Autodesk Fusion 360 part; units mm, degrees
(part 2 of 3)
sketch "Sketch24" plane through (2.9845, 0, 0) normal (1, 0, 0) x (0, 0, -1)
  circle A0 centre (17.3736, 285.75) radius 11.1125
  circle A1 centre (-17.3736, 285.75) radius 11.1125
  arc A2 (-19.05, 304.8) -> (-31.75, 292.1) centre (-19.05, 292.1) ccw
  line L0 (-31.75, 292.1) -> (-31.75, 254)
  line L1 (-31.75, 254) -> (-38.1, 254)
  line L2 (-38.1, 254) -> (-38.1, 0)
  line L3 (-38.1, 0) -> (-88.9, 0)
  line L4 (-88.9, 0) -> (-88.9, 5.969)
  line L5 (-88.9, 5.969) -> (-114.3, 5.969)
  line L6 (-114.3, 5.969) -> (-114.3, -6.35)
  arc A3 (-114.3, -6.35) -> (-101.6, -19.05) centre (-101.6, -6.35) ccw
  line L7 (-101.6, -19.05) -> (101.6, -19.05)
  arc A4 (101.6, -19.05) -> (114.3, -6.35) centre (101.6, -6.35) ccw
  line L8 (114.3, -6.35) -> (114.3, 5.969)
  line L9 (114.3, 5.969) -> (88.9, 5.969)
  line L10 (88.9, 5.969) -> (88.9, 0)
  line L11 (88.9, 0) -> (38.1, 0)
  line L12 (38.1, 0) -> (38.1, 254)
  line L13 (38.1, 254) -> (31.75, 254)
  line L14 (31.75, 254) -> (31.75, 292.1)
  arc A5 (31.75, 292.1) -> (19.05, 304.8) centre (19.05, 292.1) ccw
  line L15 (19.05, 304.8) -> (2.9845, 304.8)
  line L16 (2.9845, 304.8) -> (2.9845, -9.525)
  line L17 (2.9845, -9.525) -> (-2.9845, -9.525)
  line L18 (-2.9845, -9.525) -> (-2.9845, 304.8)
  line L19 (-2.9845, 304.8) -> (-19.05, 304.8)
  line L20 (2.9845, 304.8) -> (31.7627, 304.8) construction
  line L21 (31.7627, 304.8) -> (31.7627, 228.6) construction
  line L22 (31.7627, 228.6) -> (31.7627, 203.2) construction
  line L23 (31.7627, 203.2) -> (31.7627, 177.8) construction
  line L24 (31.7627, 177.8) -> (31.7627, 152.4) construction
  line L25 (31.7627, 152.4) -> (31.7627, 127) construction
  line L26 (31.7627, 127) -> (31.75, 101.6) construction
  line L27 (31.7627, 228.6) -> (19.0627, 228.6)
  line L28 (19.0627, 228.6) -> (19.0627, 222.631)
  line L29 (19.0627, 222.631) -> (31.7627, 222.631)
  line L30 (31.7627, 222.631) -> (31.7627, 228.6)
  line L31 (31.7627, 177.8) -> (19.0627, 177.8)
  line L32 (19.0627, 177.8) -> (19.0627, 171.831)
  line L33 (19.0627, 171.831) -> (31.7627, 171.831)
  line L34 (31.7627, 171.831) -> (31.7627, 177.8)
  line L35 (31.7627, 203.2) -> (19.0627, 203.2)
  line L36 (19.0627, 203.2) -> (19.0627, 197.231)
  line L37 (19.0627, 197.231) -> (31.7627, 197.231)
  line L38 (31.7627, 197.231) -> (31.7627, 203.2)
  line L39 (31.7627, 152.4) -> (19.0627, 152.4)
  line L40 (19.0627, 152.4) -> (19.0627, 146.431)
  line L41 (19.0627, 146.431) -> (31.7627, 146.431)
  line L42 (31.7627, 146.431) -> (31.7627, 152.4)
  line L43 (31.7627, 127) -> (19.0627, 127)
  line L44 (19.0627, 127) -> (19.0627, 121.031)
  line L45 (19.0627, 121.031) -> (31.7627, 121.031)
  line L46 (31.7627, 121.031) -> (31.7627, 127)
  line L47 (31.75, 101.6) -> (19.05, 101.6)
  line L48 (19.05, 101.6) -> (19.05, 95.631)
  line L49 (19.05, 95.631) -> (31.75, 95.631)
  line L50 (31.75, 95.631) -> (31.75, 101.6)
  dimension "d155" = 28.7782
  dimension "d156" = 76.2
  dimension "d157" = 25.4
  dimension "d158" = 25.4
  dimension "d159" = 25.4
  dimension "d160" = 25.4
  dimension "d161" = 25.4
  dimension "d162" = 12.7
  dimension "d163" = 5.969
  dimension "d164" = 12.7
  dimension "d165" = 5.969
  dimension "d166" = 12.7
  dimension "d167" = 5.969
  dimension "d168" = 12.7
  dimension "d169" = 5.969
  dimension "d170" = 12.7
  dimension "d171" = 5.969
  dimension "d172" = 12.7
  dimension "d173" = 5.969
  constraint coincident L15.end L16.start
  constraint perpendicular L16 L20
  constraint perpendicular L20 L21
  constraint parallel L14 L22
  constraint parallel L14 L23
  constraint parallel L14 L24
  constraint parallel L16 L25
  constraint coincident L14 L26.end
  constraint horizontal L27
  constraint vertical L28
  constraint horizontal L29
  constraint vertical L30
  constraint horizontal L31
  constraint vertical L32
  constraint horizontal L33
  constraint vertical L34
  constraint horizontal L35
  constraint vertical L36
  constraint horizontal L37
  constraint vertical L38
  constraint horizontal L39
  constraint vertical L40
  constraint horizontal L41
  constraint vertical L42
  constraint horizontal L43
  constraint vertical L44
  constraint horizontal L45
  constraint vertical L46
  constraint horizontal L47
  constraint vertical L48
  constraint horizontal L49
  constraint vertical L50
  measures "d155" distance of L15.end L20.end
  measures "d156" distance of L20.end L21.end
  measures "d157" distance of L21.end L22.end
  measures "d158" distance of L22.end L23.end
  measures "d159" distance of L23.end L24.end
  measures "d160" distance of L24.end L25.end
  measures "d161" distance of L25.end L26.end
  measures "d162" distance of L21.end L27.end
  measures "d163" distance of L21.end L29.end
  measures "d164" distance of L23.end L31.end
  measures "d165" distance of L23.end L33.end
  measures "d166" distance of L22.end L35.end
  measures "d167" distance of L22.end L37.end
  measures "d168" distance of L24.end L39.end
  measures "d169" distance of L24.end L41.end
  measures "d170" distance of L25.end L43.end
  measures "d171" distance of L25.end L45.end
  measures "d172" distance of L26.end L47.end
  measures "d173" distance of L26.end L49.end
sketch "Sketch25" plane through (0, 0, 0) normal (0, 1, 0) x (1, 0, 0)
  line L0 (31.369, -190.5) -> (31.369, -279.4)
  line L1 (31.369, -279.4) -> (0, -279.4)
  line L2 (0, -279.4) -> (0, -190.5)
  line L3 (12.7127, -279.4) -> (18.6817, -279.4)
  line L4 (18.6817, -203.2) -> (12.7127, -203.2)
  arc A0 (31.369, -190.5) -> (0, -190.5) centre (15.6845, -190.5) ccw
  line L5 (0, -279.4) -> (12.7, -279.4) construction
  line L6 (12.7, -279.4) -> (18.669, -279.4)
  line L7 (18.669, -279.4) -> (18.669, -203.2)
  line L8 (18.669, -203.2) -> (12.7, -203.2)
  line L9 (12.7, -203.2) -> (12.7, -279.4)
  arc A1 (0, -203.2) -> (0, -190.5) centre (-6.35, -196.85) ccw
  line L10 (0, -190.5) -> (0, -196.85) construction
  line L11 (0, -196.85) -> (2.6303, -196.85) construction
  line L12 (31.369, -190.5) -> (31.369, -196.85) construction
  line L13 (31.369, -196.85) -> (28.7274, -196.85) construction
  arc A2 (31.369, -190.5) -> (31.369, -203.2) centre (37.6804, -196.85) ccw
  line L14 (18.6817, -203.2) -> (18.6817, -225.2472) construction
  dimension "d176" = 31.369
  dimension "d177" = 88.9
  dimension "d180" = 76.2
  dimension "d185" = 12.7
  dimension "d186" = 5.969
  dimension "d187" = 76.2
  dimension "d189" = 12.7
  dimension "d190" = 6.35
  dimension "d191" = 6.35
  dimension "d192" = 2.6416
  dimension "d193" = 12.7
  dimension "d194" = 22.0472
  constraint vertical L0
  constraint horizontal L1
  constraint vertical L2
  constraint horizontal L3
  constraint horizontal L4
  constraint tangent L0 A0
  constraint perpendicular L2 L5
  constraint horizontal L6
  constraint vertical L7
  constraint horizontal L8
  constraint vertical L9
  constraint coincident L2 A1.start
  constraint parallel L2 L10
  constraint midpoint A1 L11.end
  constraint perpendicular L11 L12
  constraint perpendicular L12 L13
  constraint coincident L13.end A2
  constraint coincident L0 A2.end
  constraint perpendicular L8 L14
  measures "d176" distance of L2.end L0.start
  measures "d177" distance of L2.end L1.end
  measures "d180" distance of L3.start L4.end
  measures "d185" distance of L1.end L5.end
  measures "d186" distance of L5.end L6.end
  measures "d187" distance of L5.end L8.end
  measures "d189" distance of L2.end A1.start
  measures "d190" distance of L2.end L10.end
  measures "d191" distance of L0.start L12.end
  measures "d192" distance of L12.end L13.end
  measures "d193" distance of L0.start A2.end
  measures "d194" distance of L4.start L14.end
sketch "Sketch26" plane through (-2.9845, 0, 0) normal (-1, 0, 0) x (0, 0, 1)
  line L0 (-31.75, 254) -> (-38.1, 254)
  line L1 (-38.1, 254) -> (-38.1, 0)
  line L2 (-38.1, 0) -> (-88.9, 0)
  line L3 (-88.9, 0) -> (-88.9, 5.969)
  line L4 (-88.9, 5.969) -> (-114.3, 5.969)
  line L5 (-114.3, 5.969) -> (-114.3, -6.35)
  arc A0 (-114.3, -6.35) -> (-101.6, -19.05) centre (-101.6, -6.35) ccw
  line L6 (-101.6, -19.05) -> (101.6, -19.05)
  arc A1 (101.6, -19.05) -> (114.3, -6.35) centre (101.6, -6.35) ccw
  line L7 (114.3, -6.35) -> (114.3, 5.969)
  line L8 (114.3, 5.969) -> (88.9, 5.969)
  line L9 (88.9, 5.969) -> (88.9, 0)
  line L10 (88.9, 0) -> (38.1, 0)
  line L11 (38.1, 0) -> (38.1, 254)
  line L12 (38.1, 254) -> (31.75, 254)
  line L13 (31.75, 254) -> (31.75, 292.1)
  arc A2 (31.75, 292.1) -> (19.05, 304.8) centre (19.05, 292.1) ccw
  line L14 (19.05, 304.8) -> (2.9845, 304.8)
  line L15 (2.9845, 304.8) -> (2.9845, -9.525)
  line L16 (2.9845, -9.525) -> (-2.9845, -9.525)
  line L17 (-2.9845, -9.525) -> (-2.9845, 304.8)
  line L18 (-2.9845, 304.8) -> (-19.05, 304.8)
  arc A3 (-19.05, 304.8) -> (-31.75, 292.1) centre (-19.05, 292.1) ccw
  line L19 (-31.75, 292.1) -> (-31.75, 254)
  circle A4 centre (17.3736, 285.75) radius 11.1125
  circle A5 centre (-17.3736, 285.75) radius 11.1125
sketch "Sketch27" plane through (0, 0, 2.9845) normal (0, 0, 1) x (1, 0, 0)
  circle A0 centre (17.3609, 285.75) radius 11.1125
  circle A1 centre (-17.3609, 285.75) radius 11.1125
  arc A2 (-19.05, 304.8) -> (-31.75, 292.1) centre (-19.05, 292.1) ccw
  line L0 (-31.75, 292.1) -> (-31.75, 254)
  line L1 (-31.75, 254) -> (-38.1, 254)
  line L2 (-38.1, 254) -> (-38.1, 0)
  line L3 (-38.1, 0) -> (-88.9, 0)
  line L4 (-88.9, 0) -> (-88.9, 5.969)
  line L5 (-88.9, 5.969) -> (-114.3, 5.969)
  line L6 (-114.3, 5.969) -> (-114.3, -6.35)
  arc A3 (-114.3, -6.35) -> (-101.6, -19.05) centre (-101.6, -6.35) ccw
  line L7 (-101.6, -19.05) -> (-2.9845, -19.05)
  line L8 (-2.9845, -19.05) -> (-2.9845, -9.525)
  line L9 (-2.9845, -9.525) -> (2.9845, -9.525)
  line L10 (2.9845, -9.525) -> (2.9845, -19.05)
  line L11 (2.9845, -19.05) -> (101.6, -19.05)
  arc A4 (101.6, -19.05) -> (114.3, -6.35) centre (101.6, -6.35) ccw
  line L12 (114.3, -6.35) -> (114.3, 5.969)
  line L13 (114.3, 5.969) -> (88.9, 5.969)
  line L14 (88.9, 5.969) -> (88.9, 0)
  line L15 (88.9, 0) -> (38.1, 0)
  line L16 (38.1, 0) -> (38.1, 254)
  line L17 (38.1, 254) -> (31.75, 254)
  line L18 (31.75, 254) -> (31.75, 292.1)
  arc A5 (31.75, 292.1) -> (19.05, 304.8) centre (19.05, 292.1) ccw
  line L19 (19.05, 304.8) -> (-19.05, 304.8)
sketch "Sketch28" plane through (0, 5.969, 0) normal (0, 1, 0) x (-1, 0, 0)
  arc A0 (-495.3, 367.5922) -> (-596.1922, 266.7) centre (-482.6, 254) ccw
  line L0 (-596.1922, 266.7) -> (-602.5797, 266.7)
  arc A1 (-495.3, 373.9797) -> (-602.5797, 266.7) centre (-482.6, 254) ccw
  line L1 (-495.3, 373.9797) -> (-495.3, 367.5922)
  arc A2 (-469.9, 166.0118) -> (-394.6118, 241.3) centre (-482.6, 254) ccw
  line L2 (-394.6118, 241.3) -> (-388.2005, 241.3)
  arc A3 (-469.9, 159.6005) -> (-388.2005, 241.3) centre (-482.6, 254) ccw
  line L3 (-469.9, 159.6005) -> (-469.9, 166.0118)
  arc A4 (-420.383, 266.7) -> (-469.9, 316.217) centre (-482.6, 254) ccw
  line L4 (-469.9, 316.217) -> (-469.9, 322.6857)
  arc A5 (-413.9142, 266.7) -> (-469.9, 322.6857) centre (-482.6, 254) ccw
  line L5 (-413.9142, 266.7) -> (-420.383, 266.7)
  arc A6 (-469.9, 191.783) -> (-420.383, 241.3) centre (-482.6, 254) ccw
  line L6 (-420.383, 241.3) -> (-413.9142, 241.3)
  arc A7 (-469.9, 185.3142) -> (-413.9142, 241.3) centre (-482.6, 254) ccw
  line L7 (-469.9, 185.3142) -> (-469.9, 191.783)
  arc A8 (-394.6118, 266.7) -> (-469.9, 341.9882) centre (-482.6, 254) ccw
  line L8 (-469.9, 341.9882) -> (-469.9, 348.3995)
  arc A9 (-388.2005, 266.7) -> (-469.9, 348.3995) centre (-482.6, 254) ccw
  line L9 (-388.2005, 266.7) -> (-394.6118, 266.7)
  arc A10 (-469.9, 140.4077) -> (-369.0077, 241.3) centre (-482.6, 254) ccw
  line L10 (-369.0077, 241.3) -> (-362.6203, 241.3)
  arc A11 (-469.9, 134.0203) -> (-362.6203, 241.3) centre (-482.6, 254) ccw
  line L11 (-469.9, 134.0203) -> (-469.9, 140.4077)
  arc A12 (-369.0077, 266.7) -> (-469.9, 367.5922) centre (-482.6, 254) ccw
  line L12 (-469.9, 367.5922) -> (-469.9, 373.9797)
  arc A13 (-362.6203, 266.7) -> (-469.9, 373.9797) centre (-482.6, 254) ccw
  line L13 (-362.6203, 266.7) -> (-369.0077, 266.7)
  arc A14 (-570.5882, 241.3) -> (-495.3, 166.0118) centre (-482.6, 254) ccw
  line L14 (-495.3, 166.0118) -> (-495.3, 159.6005)
  arc A15 (-576.9995, 241.3) -> (-495.3, 159.6005) centre (-482.6, 254) ccw
  line L15 (-576.9995, 241.3) -> (-570.5882, 241.3)
  arc A16 (-495.3, 316.217) -> (-544.817, 266.7) centre (-482.6, 254) ccw
  line L16 (-544.817, 266.7) -> (-551.2857, 266.7)
  arc A17 (-495.3, 322.6857) -> (-551.2857, 266.7) centre (-482.6, 254) ccw
  line L17 (-495.3, 322.6857) -> (-495.3, 316.217)
  arc A18 (-544.817, 241.3) -> (-495.3, 191.783) centre (-482.6, 254) ccw
  line L18 (-495.3, 191.783) -> (-495.3, 185.3142)
  arc A19 (-551.2857, 241.3) -> (-495.3, 185.3142) centre (-482.6, 254) ccw
  line L19 (-551.2857, 241.3) -> (-544.817, 241.3)
  arc A20 (-495.3, 341.9882) -> (-570.5882, 266.7) centre (-482.6, 254) ccw
  line L20 (-570.5882, 266.7) -> (-576.9995, 266.7)
  arc A21 (-495.3, 348.3995) -> (-576.9995, 266.7) centre (-482.6, 254) ccw
  line L21 (-495.3, 348.3995) -> (-495.3, 341.9882)
  arc A22 (-596.1922, 241.3) -> (-495.3, 140.4077) centre (-482.6, 254) ccw
  line L22 (-495.3, 140.4077) -> (-495.3, 134.0203)
  arc A23 (-602.5797, 241.3) -> (-495.3, 134.0203) centre (-482.6, 254) ccw
  line L23 (-602.5797, 241.3) -> (-596.1922, 241.3)
  line L24 (-485.5845, 251.0155) -> (-514.35, 251.0155)
  line L25 (-514.35, 251.0155) -> (-514.35, 256.9845)
  line L26 (-514.35, 256.9845) -> (-485.5845, 256.9845)
  line L27 (-485.5845, 256.9845) -> (-485.5845, 285.75)
  line L28 (-485.5845, 285.75) -> (-479.6155, 285.75)
  line L29 (-479.6155, 285.75) -> (-479.6155, 256.9845)
  line L30 (-479.6155, 256.9845) -> (-450.85, 256.9845)
  line L31 (-450.85, 256.9845) -> (-450.85, 251.0155)
  line L32 (-450.85, 251.0155) -> (-479.6155, 251.0155)
  line L33 (-479.6155, 251.0155) -> (-479.6155, 222.25)
  line L34 (-479.6155, 222.25) -> (-485.5845, 222.25)
  line L35 (-485.5845, 222.25) -> (-485.5845, 251.0155)
  circle A24 centre (-482.6, 254) radius 152.4
  line L36 (-479.6155, 251.0155) -> (-457.1649, 228.5648) construction
  line L37 (-485.5845, 256.9845) -> (-508.0351, 279.4351) construction
  line L38 (-485.5845, 251.0155) -> (-508.0351, 228.5649) construction
  line L39 (-485.5845, 251.0155) -> (-453.8345, 251.0155) construction
  line L40 (-479.6155, 256.9845) -> (-457.1649, 279.4351) construction
  line L41 (-479.6155, 256.9845) -> (-447.8655, 256.9845) construction
  line L42 (-485.5845, 222.25) -> (-485.5845, 215.265)
  line L43 (-450.85, 251.0155) -> (-449.58, 251.0155)
  line L44 (-449.58, 251.0155) -> (-442.595, 251.0155)
  line L45 (-479.6155, 285.75) -> (-479.6155, 292.735)
  line L46 (-514.35, 256.9845) -> (-521.335, 256.9845)
  line L47 (-514.35, 251.0155) -> (-511.175, 251.0155)
  line L48 (-485.5845, 285.75) -> (-485.5845, 282.575)
  line L49 (-450.85, 256.9845) -> (-454.025, 256.9845)
  line L50 (-479.6155, 222.25) -> (-479.6155, 225.425)
  arc A25 (-479.6155, 225.425) -> (-442.595, 251.0155) centre (-472.206, 254.2792) ccw
  arc A26 (-511.175, 251.0155) -> (-485.5845, 215.265) centre (-484.108, 243.3561) ccw
  arc A27 (-485.5845, 282.575) -> (-521.335, 256.9845) centre (-493.2439, 255.508) ccw
  arc A28 (-454.025, 256.9845) -> (-479.6155, 292.735) centre (-481.092, 264.6439) ccw
  line L51 (-442.595, 251.0155) -> (-442.595, 256.9845)
  line L52 (-442.595, 256.9845) -> (-454.025, 256.9845)
  line L53 (-479.6155, 292.735) -> (-485.5845, 292.735)
  line L54 (-485.5845, 292.735) -> (-485.5845, 282.575)
  line L55 (-521.335, 256.9845) -> (-521.335, 251.0155)
  line L56 (-521.335, 251.0155) -> (-511.175, 251.0155)
  line L57 (-485.5845, 215.265) -> (-479.6155, 215.265)
  line L58 (-479.6155, 215.265) -> (-479.6155, 225.425)
  dimension "d314" = 31.75
  dimension "d315" = 31.75
  dimension "d316" = 135
  dimension "d317" = 31.75
  dimension "d320" = 45
  dimension "d321" = 31.75
  dimension "d327" = 6.985
  dimension "d328" = 6.985
  dimension "d329" = 6.985
  dimension "d330" = 6.985
  dimension "d331" = 3.175
  dimension "d332" = 3.175
  dimension "d333" = 3.175
  dimension "d334" = 3.175
  dimension "d335" = 5.969
  dimension "d336" = 5.969
  constraint coincident L29.end L30.start
  constraint coincident L32.end L33.start
  constraint coincident L26.end L27.start
  constraint horizontal L39
  constraint coincident L24.start L35.end
  constraint horizontal L41
  constraint coincident L34.end L35.start
  constraint perpendicular L34 L42
  constraint coincident L31.end L32.start
  constraint perpendicular L31 L43
  constraint perpendicular L31 L44
  constraint coincident L28.end L29.start
  constraint perpendicular L28 L45
  constraint coincident L25.end L26.start
  constraint perpendicular L25 L46
  constraint coincident L24.end L25.start
  constraint perpendicular L25 L47
  constraint coincident L27.end L28.start
  constraint perpendicular L28 L48
  constraint coincident L30.end L31.start
  constraint perpendicular L31 L49
  constraint coincident L33.end L34.start
  constraint perpendicular L34 L50
  constraint coincident L36.end A25
  constraint coincident L38.end A26
  constraint coincident L37.end A27
  constraint coincident L40.end A28
  constraint perpendicular L44 L51
  constraint perpendicular L45 L53
  constraint perpendicular L53 L54
  constraint perpendicular L46 L55
  constraint perpendicular L55 L56
  constraint perpendicular L42 L57
  measures "d314" distance of L32.end L36.end
  measures "d315" distance of L26.end L37.end
  measures "d316" angle of L38 L39
  measures "d317" distance of L24.start L38.end
  measures "d320" angle of L40 L41
  measures "d321" distance of L29.end L40.end
  measures "d327" distance of L34.end L42.end
  measures "d328" distance of L43.end L44.end
  measures "d329" distance of L28.end L45.end
  measures "d330" distance of L25.end L46.end
  measures "d331" distance of L24.end L47.end
  measures "d332" distance of L27.end L48.end
  measures "d333" distance of L30.end L49.end
  measures "d334" distance of L33.end L50.end
  measures "d335" distance of L44.end L51.end
  measures "d336" distance of L42.end L57.end
extrude "Extrude3'''" cut sketch "Sketch28" against normal up to surface (5.969 mm away) contours L24 L35 L42 A26 | L34 L42 L57 L58 | L25 L46 L55 L56 | L26 L27 L46 A27 | L32 L33 L43 L44 A25 | L31 L43 L44 L51 L52 | L28 L45 L53 L54 | L29 L30 L45 A28 bodies 6 in component "Component'''"
extrude "Extrude2''''" cut sketch "Sketch28" against normal up to surface (5.969 mm away) contours L24 L25 L26 L27 L28 L29 L30 L31 L32 L33 L34 L35 L47 L48 L49 L50 L52 L54 L56 L58 | L28 L45 L53 L54 | L29 L30 L45 A28 bodies 6 in component "Component'''"
extrude "Extrude1''''" cut sketch "Sketch28" against normal up to surface (5.969 mm away) contours L24 L35 L42 A26 | L24 L25 L26 L27 L28 L29 L30 L31 L32 L33 L34 L35 L47 L48 L49 L50 L52 L54 L56 L58 | L26 L27 L46 A27 | L32 L33 L43 L44 A25 | L29 L30 L45 A28 bodies 6 in component "Component'''"
sketch "Sketch29" plane through (0, 0, 2.9845) normal (0, 0, 1) x (1, 0, 0)
  circle A0 centre (17.3609, 285.75) radius 11.1125
  circle A1 centre (-17.3609, 285.75) radius 11.1125
  arc A2 (-19.05, 304.8) -> (-31.75, 292.1) centre (-19.05, 292.1) ccw
  line L0 (-31.75, 292.1) -> (-31.75, 254)
  line L1 (-31.75, 254) -> (-38.1, 254)
  line L2 (-38.1, 254) -> (-38.1, 0)
  line L3 (-38.1, 0) -> (-88.9, 0)
  line L4 (-88.9, 0) -> (-88.9, 5.969)
  line L5 (-88.9, 5.969) -> (-114.3, 5.969)
  line L6 (-114.3, 5.969) -> (-114.3, -6.35)
  arc A3 (-114.3, -6.35) -> (-101.6, -19.05) centre (-101.6, -6.35) ccw
  line L7 (-101.6, -19.05) -> (-2.9845, -19.05)
  line L8 (-2.9845, -19.05) -> (-2.9845, -9.525)
  line L9 (-2.9845, -9.525) -> (2.9845, -9.525)
  line L10 (2.9845, -9.525) -> (2.9845, -19.05)
  line L11 (2.9845, -19.05) -> (101.6, -19.05)
  arc A4 (101.6, -19.05) -> (114.3, -6.35) centre (101.6, -6.35) ccw
  line L12 (114.3, -6.35) -> (114.3, 5.969)
  line L13 (114.3, 5.969) -> (88.9, 5.969)
  line L14 (88.9, 5.969) -> (88.9, 0)
  line L15 (88.9, 0) -> (38.1, 0)
  line L16 (38.1, 0) -> (38.1, 254)
  line L17 (38.1, 254) -> (31.75, 254)
  line L18 (31.75, 254) -> (31.75, 292.1)
  arc A5 (31.75, 292.1) -> (19.05, 304.8) centre (19.05, 292.1) ccw
  line L19 (19.05, 304.8) -> (-19.05, 304.8)
  line L20 (38.1, 254) -> (38.1, 228.6) construction
  line L21 (38.1, 228.6) -> (38.1, 203.2) construction
  line L22 (38.1, 203.2) -> (38.1, 177.8) construction
  line L23 (38.1, 177.8) -> (38.1, 152.4) construction
  line L24 (38.1, 152.4) -> (38.1, 127) construction
  line L25 (38.1, 127) -> (38.1, 101.6) construction
  line L26 (38.1, 101.6) -> (38.1, 76.2) construction
  line L27 (38.1, 76.2) -> (38.1, 50.8) construction
  line L28 (-38.1, 254) -> (-38.1, 228.6) construction
  line L29 (-38.1, 228.6) -> (-38.1, 203.2) construction
  line L30 (-38.1, 203.2) -> (-38.1, 177.8) construction
  line L31 (-38.1, 177.8) -> (-38.1, 152.4) construction
  line L32 (-38.1, 152.4) -> (-38.1, 127) construction
  line L33 (-38.1, 127) -> (-38.1, 101.6) construction
  line L34 (-38.1, 101.6) -> (-38.1, 76.2) construction
  line L35 (-38.1, 76.2) -> (-38.1, 50.8) construction
  line L36 (-38.1, 228.6) -> (-32.131, 228.6)
  line L37 (-32.131, 228.6) -> (-32.131, 222.631)
  line L38 (-32.131, 222.631) -> (-38.1, 222.631)
  line L39 (-38.1, 222.631) -> (-38.1, 228.6)
  line L40 (-38.1, 203.2) -> (-32.131, 203.2)
  line L41 (-32.131, 203.2) -> (-32.131, 197.231)
  line L42 (-32.131, 197.231) -> (-38.1, 197.231)
  line L43 (-38.1, 197.231) -> (-38.1, 203.2)
  line L44 (-38.1, 177.8) -> (-32.131, 177.8)
  line L45 (-32.131, 177.8) -> (-32.131, 171.831)
  line L46 (-32.131, 171.831) -> (-38.1, 171.831)
  line L47 (-38.1, 171.831) -> (-38.1, 177.8)
  line L48 (-38.1, 152.4) -> (-32.131, 152.4)
  line L49 (-32.131, 152.4) -> (-32.131, 146.431)
  line L50 (-32.131, 146.431) -> (-38.1, 146.431)
  line L51 (-38.1, 146.431) -> (-38.1, 152.4)
  line L52 (-38.1, 127) -> (-32.131, 127)
  line L53 (-32.131, 127) -> (-32.131, 121.031)
  line L54 (-32.131, 121.031) -> (-38.1, 121.031)
  line L55 (-38.1, 121.031) -> (-38.1, 127)
  line L56 (-38.1, 101.6) -> (-32.131, 101.6)
  line L57 (-32.131, 101.6) -> (-32.131, 95.631)
  line L58 (-32.131, 95.631) -> (-38.1, 95.631)
  line L59 (-38.1, 95.631) -> (-38.1, 101.6)
  line L60 (-38.1, 76.2) -> (-32.131, 76.2)
  line L61 (-32.131, 76.2) -> (-32.131, 70.231)
  line L62 (-32.131, 70.231) -> (-38.1, 70.231)
  line L63 (-38.1, 70.231) -> (-38.1, 76.2)
  line L64 (-38.1, 50.8) -> (-32.131, 50.8)
  line L65 (-32.131, 50.8) -> (-32.131, 44.831)
  line L66 (-32.131, 44.831) -> (-38.1, 44.831)
  line L67 (-38.1, 44.831) -> (-38.1, 50.8)
  line L68 (38.1, 50.8) -> (32.131, 50.8)
  line L69 (32.131, 50.8) -> (32.131, 44.831)
  line L70 (32.131, 44.831) -> (38.1, 44.831)
  line L71 (38.1, 44.831) -> (38.1, 50.8)
  line L72 (38.1, 76.2) -> (32.131, 76.2)
  line L73 (32.131, 76.2) -> (32.131, 70.231)
  line L74 (32.131, 70.231) -> (38.1, 70.231)
  line L75 (38.1, 70.231) -> (38.1, 76.2)
  line L76 (38.1, 101.6) -> (32.131, 101.6)
  line L77 (32.131, 101.6) -> (32.131, 95.631)
  line L78 (32.131, 95.631) -> (38.1, 95.631)
  line L79 (38.1, 95.631) -> (38.1, 101.6)
  line L80 (38.1, 127) -> (32.131, 127)
  line L81 (32.131, 127) -> (32.131, 121.031)
  line L82 (32.131, 121.031) -> (38.1, 121.031)
  line L83 (38.1, 121.031) -> (38.1, 127)
  line L84 (38.1, 152.4) -> (32.131, 152.4)
  line L85 (32.131, 152.4) -> (32.131, 146.431)
  line L86 (32.131, 146.431) -> (38.1, 146.431)
  line L87 (38.1, 146.431) -> (38.1, 152.4)
  line L88 (38.1, 177.8) -> (32.131, 177.8)
  line L89 (32.131, 177.8) -> (32.131, 171.831)
  line L90 (32.131, 171.831) -> (38.1, 171.831)
  line L91 (38.1, 171.831) -> (38.1, 177.8)
  line L92 (38.1, 203.2) -> (32.131, 203.2)
  line L93 (32.131, 203.2) -> (32.131, 197.231)
  line L94 (32.131, 197.231) -> (38.1, 197.231)
  line L95 (38.1, 197.231) -> (38.1, 203.2)
  line L96 (38.1, 228.6) -> (32.131, 228.6)
  line L97 (32.131, 228.6) -> (32.131, 222.631)
  line L98 (32.131, 222.631) -> (38.1, 222.631)
  line L99 (38.1, 222.631) -> (38.1, 228.6)
  dimension "d206" = 25.4
  dimension "d207" = 25.4
  dimension "d208" = 25.4
  dimension "d209" = 25.4
  dimension "d210" = 25.4
  dimension "d211" = 25.4
  dimension "d212" = 25.4
  dimension "d213" = 25.4
  dimension "d214" = 25.4
  dimension "d215" = 25.4
  dimension "d216" = 25.4
  dimension "d217" = 25.4
  dimension "d218" = 25.4
  dimension "d219" = 25.4
  dimension "d220" = 25.4
  dimension "d221" = 25.4
  dimension "d222" = 5.969
  dimension "d223" = 5.969
  dimension "d224" = 5.969
  dimension "d225" = 5.969
  dimension "d226" = 5.969
  dimension "d227" = 5.969
  dimension "d228" = 5.969
  dimension "d229" = 5.969
  dimension "d230" = 5.969
  dimension "d231" = 5.969
  dimension "d232" = 5.969
  dimension "d233" = 5.969
  dimension "d234" = 5.969
  dimension "d235" = 5.969
  dimension "d236" = 5.969
  dimension "d237" = 5.969
  dimension "d238" = 5.969
  dimension "d239" = 5.969
  dimension "d240" = 5.969
  dimension "d241" = 5.969
  dimension "d242" = 5.969
  dimension "d243" = 5.969
  dimension "d244" = 5.969
  dimension "d245" = 5.969
  dimension "d246" = 5.969
  dimension "d247" = 5.969
  dimension "d248" = 5.969
  dimension "d249" = 5.969
  dimension "d250" = 5.969
  dimension "d251" = 5.969
  dimension "d252" = 5.969
  dimension "d253" = 5.969
  constraint coincident L16.end L17.start
  constraint perpendicular L17 L20
  constraint parallel L16 L21
  constraint parallel L16 L22
  constraint parallel L16 L23
  constraint parallel L16 L24
  constraint parallel L16 L25
  constraint parallel L16 L26
  constraint parallel L16 L27
  constraint coincident L1.end L2.start
  constraint perpendicular L1 L28
  constraint parallel L2 L29
  constraint parallel L2 L30
  constraint parallel L2 L31
  constraint parallel L2 L32
  constraint parallel L2 L33
  constraint parallel L2 L34
  constraint parallel L2 L35
  constraint horizontal L36
  constraint vertical L37
  constraint horizontal L38
  constraint vertical L39
  constraint horizontal L40
  constraint vertical L41
  constraint horizontal L42
  constraint vertical L43
  constraint horizontal L44
  constraint vertical L45
  constraint horizontal L46
  constraint vertical L47
  constraint horizontal L48
  constraint vertical L49
  constraint horizontal L50
  constraint vertical L51
  constraint horizontal L52
  constraint vertical L53
  constraint horizontal L54
  constraint vertical L55
  constraint horizontal L56
  constraint vertical L57
  constraint horizontal L58
  constraint vertical L59
  constraint horizontal L60
  constraint vertical L61
  constraint horizontal L62
  constraint vertical L63
  constraint horizontal L64
  constraint vertical L65
  constraint horizontal L66
  constraint vertical L67
  constraint horizontal L68
  constraint vertical L69
  constraint horizontal L70
  constraint vertical L71
  constraint horizontal L72
  constraint vertical L73
  constraint horizontal L74
  constraint vertical L75
  constraint horizontal L76
  constraint vertical L77
  constraint horizontal L78
  constraint vertical L79
  constraint horizontal L80
  constraint vertical L81
  constraint horizontal L82
  constraint vertical L83
  constraint horizontal L84
  constraint vertical L85
  constraint horizontal L86
  constraint vertical L87
  constraint horizontal L88
  constraint vertical L89
  constraint horizontal L90
  constraint vertical L91
  constraint horizontal L92
  constraint vertical L93
  constraint horizontal L94
  constraint vertical L95
  constraint horizontal L96
  constraint vertical L97
  constraint horizontal L98
  constraint vertical L99
  measures "d206" distance of L16.end L20.end
  measures "d207" distance of L20.end L21.end
  measures "d208" distance of L21.end L22.end
  measures "d209" distance of L22.end L23.end
  measures "d210" distance of L23.end L24.end
  measures "d211" distance of L24.end L25.end
  measures "d212" distance of L25.end L26.end
  measures "d213" distance of L26.end L27.end
  measures "d214" distance of L1.end L28.end
  measures "d215" distance of L28.end L29.end
  measures "d216" distance of L29.end L30.end
  measures "d217" distance of L30.end L31.end
  measures "d218" distance of L31.end L32.end
  measures "d219" distance of L32.end L33.end
  measures "d220" distance of L33.end L34.end
  measures "d221" distance of L34.end L35.end
  measures "d222" distance of L28.end L36.end
  measures "d223" distance of L28.end L38.end
  measures "d224" distance of L29.end L40.end
  measures "d225" distance of L29.end L42.end
  measures "d226" distance of L30.end L44.end
  measures "d227" distance of L30.end L46.end
  measures "d228" distance of L31.end L48.end
  measures "d229" distance of L31.end L50.end
  measures "d230" distance of L32.end L52.end
  measures "d231" distance of L32.end L54.end
  measures "d232" distance of L33.end L56.end
  measures "d233" distance of L33.end L58.end
  measures "d234" distance of L34.end L60.end
  measures "d235" distance of L34.end L62.end
  measures "d236" distance of L35.end L64.end
  measures "d237" distance of L35.end L66.end
  measures "d238" distance of L27.end L68.end
  measures "d239" distance of L27.end L70.end
  measures "d240" distance of L26.end L72.end
  measures "d241" distance of L26.end L74.end
  measures "d242" distance of L25.end L76.end
  measures "d243" distance of L25.end L78.end
  measures "d244" distance of L24.end L80.end
  measures "d245" distance of L24.end L82.end
  measures "d246" distance of L23.end L84.end
  measures "d247" distance of L23.end L86.end
  measures "d248" distance of L22.end L88.end
  measures "d249" distance of L22.end L90.end
  measures "d250" distance of L21.end L92.end
  measures "d251" distance of L21.end L94.end
  measures "d252" distance of L20.end L96.end
  measures "d253" distance of L20.end L98.end
extrude "Extrude7'" cut sketch "Sketch29" against normal up to surface (5.969 mm away) contours L2 L36 L37 L38 L39 | L16 L96 L97 L98 L99 | L2 L40 L41 L42 L43 | L16 L92 L93 L94 L95 | L2 L44 L45 L46 L47 | L16 L88 L89 L90 L91 | L2 L48 L49 L50 L51 | L16 L84 L85 L86 L87 | L2 L52 L53 L54 L55 | L16 L80 L81 L82 L83 | L2 L56 L57 L58 L59 | L16 L76 L77 L78 L79 | L2 L60 L61 L62 L63 | L16 L72 L73 L74 L75 | L2 L64 L65 L66 L67 | L16 L68 L69 L70 L71 bodies 3 in component "Component'"
sketch "Sketch30" plane through (2.9845, 0, 0) normal (1, 0, 0) x (0, 0, -1)
  circle A0 centre (17.3736, 285.75) radius 11.1125
  circle A1 centre (-17.3736, 285.75) radius 11.1125
  arc A2 (-19.05, 304.8) -> (-31.75, 292.1) centre (-19.05, 292.1) ccw
  line L0 (-31.75, 292.1) -> (-31.75, 254)
  line L1 (-31.75, 254) -> (-38.1, 254)
  line L2 (-38.1, 254) -> (-38.1, 0)
  line L3 (-38.1, 0) -> (-88.9, 0)
  line L4 (-88.9, 0) -> (-88.9, 5.969)
  line L5 (-88.9, 5.969) -> (-114.3, 5.969)
  line L6 (-114.3, 5.969) -> (-114.3, -6.35)
  arc A3 (-114.3, -6.35) -> (-101.6, -19.05) centre (-101.6, -6.35) ccw
  line L7 (-101.6, -19.05) -> (101.6, -19.05)
  arc A4 (101.6, -19.05) -> (114.3, -6.35) centre (101.6, -6.35) ccw
  line L8 (114.3, -6.35) -> (114.3, 5.969)
  line L9 (114.3, 5.969) -> (88.9, 5.969)
  line L10 (88.9, 5.969) -> (88.9, 0)
  line L11 (88.9, 0) -> (38.1, 0)
  line L12 (38.1, 0) -> (38.1, 254)
  line L13 (38.1, 254) -> (31.75, 254)
  line L14 (31.75, 254) -> (31.75, 292.1)
  arc A5 (31.75, 292.1) -> (19.05, 304.8) centre (19.05, 292.1) ccw
  line L15 (19.05, 304.8) -> (2.9845, 304.8)
  line L16 (2.9845, 304.8) -> (2.9845, -9.525)
  line L17 (2.9845, -9.525) -> (-2.9845, -9.525)
  line L18 (-2.9845, -9.525) -> (-2.9845, 304.8)
  line L19 (-2.9845, 304.8) -> (-19.05, 304.8)
  line L20 (38.1, 254) -> (38.1, 228.6) construction
  line L21 (38.1, 228.6) -> (38.1, 203.2) construction
  line L22 (38.1, 203.2) -> (38.1, 177.8) construction
  line L23 (38.1, 177.8) -> (38.1, 152.4) construction
  line L24 (38.1, 152.4) -> (38.1, 127) construction
  line L25 (38.1, 127) -> (38.1, 101.6) construction
  line L26 (38.1, 101.6) -> (38.1, 76.2) construction
  line L27 (38.1, 76.2) -> (38.1, 50.8) construction
  line L28 (-38.1, 254) -> (-38.1, 228.6) construction
  line L29 (-38.1, 228.6) -> (-38.1, 203.2) construction
  line L30 (-38.1, 203.2) -> (-38.1, 177.8) construction
  line L31 (-38.1, 177.8) -> (-38.1, 152.4) construction
  line L32 (-38.1, 152.4) -> (-38.1, 127) construction
  line L33 (-38.1, 127) -> (-38.1, 101.6) construction
  line L34 (-38.1, 101.6) -> (-38.1, 76.2) construction
  line L35 (-38.1, 76.2) -> (-38.1, 50.8) construction
  line L36 (-38.1, 228.6) -> (-32.131, 228.6)
  line L37 (-32.131, 228.6) -> (-32.131, 222.631)
  line L38 (-32.131, 222.631) -> (-38.1, 222.631)
  line L39 (-38.1, 222.631) -> (-38.1, 228.6)
  line L40 (-38.1, 203.2) -> (-32.131, 203.2)
  line L41 (-32.131, 203.2) -> (-32.131, 197.231)
  line L42 (-32.131, 197.231) -> (-38.1, 197.231)
  line L43 (-38.1, 197.231) -> (-38.1, 203.2)
  line L44 (-38.1, 177.8) -> (-32.131, 177.8)
  line L45 (-32.131, 177.8) -> (-32.131, 171.831)
  line L46 (-32.131, 171.831) -> (-38.1, 171.831)
  line L47 (-38.1, 171.831) -> (-38.1, 177.8)
  line L48 (-38.1, 152.4) -> (-32.131, 152.4)
  line L49 (-32.131, 152.4) -> (-32.131, 146.431)
  line L50 (-32.131, 146.431) -> (-38.1, 146.431)
  line L51 (-38.1, 146.431) -> (-38.1, 152.4)
  line L52 (-38.1, 127) -> (-32.131, 127)
  line L53 (-32.131, 127) -> (-32.131, 121.031)
  line L54 (-32.131, 121.031) -> (-38.1, 121.031)
  line L55 (-38.1, 121.031) -> (-38.1, 127)
  line L56 (-38.1, 101.6) -> (-32.131, 101.6)
  line L57 (-32.131, 101.6) -> (-32.131, 95.631)
  line L58 (-32.131, 95.631) -> (-38.1, 95.631)
  line L59 (-38.1, 95.631) -> (-38.1, 101.6)
  line L60 (-38.1, 50.8) -> (-32.131, 50.8)
  line L61 (-32.131, 50.8) -> (-32.131, 44.831)
  line L62 (-32.131, 44.831) -> (-38.1, 44.831)
  line L63 (-38.1, 44.831) -> (-38.1, 50.8)
  line L64 (-38.1, 76.2) -> (-32.131, 76.2)
  line L65 (-32.131, 76.2) -> (-32.131, 70.231)
  line L66 (-32.131, 70.231) -> (-38.1, 70.231)
  line L67 (-38.1, 70.231) -> (-38.1, 76.2)
  line L68 (38.1, 50.8) -> (32.131, 50.8)
  line L69 (32.131, 50.8) -> (32.131, 44.831)
  line L70 (32.131, 44.831) -> (38.1, 44.831)
  line L71 (38.1, 44.831) -> (38.1, 50.8)
  line L72 (38.1, 76.2) -> (32.131, 76.2)
  line L73 (32.131, 76.2) -> (32.131, 70.231)
  line L74 (32.131, 70.231) -> (38.1, 70.231)
  line L75 (38.1, 70.231) -> (38.1, 76.2)
  line L76 (38.1, 101.6) -> (32.131, 101.6)
  line L77 (32.131, 101.6) -> (32.131, 95.631)
  line L78 (32.131, 95.631) -> (38.1, 95.631)
  line L79 (38.1, 95.631) -> (38.1, 101.6)
  line L80 (38.1, 127) -> (32.131, 127)
  line L81 (32.131, 127) -> (32.131, 121.031)
  line L82 (32.131, 121.031) -> (38.1, 121.031)
  line L83 (38.1, 121.031) -> (38.1, 127)
  line L84 (38.1, 152.4) -> (32.131, 152.4)
  line L85 (32.131, 152.4) -> (32.131, 146.431)
  line L86 (32.131, 146.431) -> (38.1, 146.431)
  line L87 (38.1, 146.431) -> (38.1, 152.4)
  line L88 (38.1, 177.8) -> (32.131, 177.8)
  line L89 (32.131, 177.8) -> (32.131, 171.831)
  line L90 (32.131, 171.831) -> (38.1, 171.831)
  line L91 (38.1, 171.831) -> (38.1, 177.8)
  line L92 (38.1, 203.2) -> (32.131, 203.2)
  line L93 (32.131, 203.2) -> (32.131, 197.231)
  line L94 (32.131, 197.231) -> (38.1, 197.231)
  line L95 (38.1, 197.231) -> (38.1, 203.2)
  line L96 (38.1, 228.6) -> (32.131, 228.6)
  line L97 (32.131, 228.6) -> (32.131, 222.631)
  line L98 (32.131, 222.631) -> (38.1, 222.631)
  line L99 (38.1, 222.631) -> (38.1, 228.6)
  dimension "d256" = 25.4
  dimension "d257" = 25.4
  dimension "d258" = 25.4
  dimension "d259" = 25.4
  dimension "d260" = 25.4
  dimension "d261" = 25.4
  dimension "d262" = 25.4
  dimension "d263" = 25.4
  dimension "d264" = 25.4
  dimension "d265" = 25.4
  dimension "d266" = 25.4
  dimension "d267" = 25.4
  dimension "d268" = 25.4
  dimension "d269" = 25.4
  dimension "d270" = 25.4
  dimension "d271" = 5.969
  dimension "d272" = 5.969
  dimension "d273" = 5.969
  dimension "d274" = 5.969
  dimension "d275" = 5.969
  dimension "d276" = 5.969
  dimension "d277" = 5.969
  dimension "d278" = 5.969
  dimension "d279" = 5.969
  dimension "d280" = 5.969
  dimension "d281" = 5.969
  dimension "d282" = 5.969
  dimension "d283" = 5.969
  dimension "d284" = 5.969
  dimension "d285" = 5.969
  dimension "d286" = 5.969
  dimension "d287" = 5.969
  dimension "d288" = 5.969
  dimension "d289" = 5.969
  dimension "d290" = 5.969
  dimension "d291" = 5.969
  dimension "d292" = 5.969
  dimension "d293" = 5.969
  dimension "d294" = 5.969
  dimension "d295" = 5.969
  dimension "d296" = 5.969
  dimension "d297" = 5.969
  dimension "d298" = 5.969
  dimension "d299" = 5.969
  dimension "d300" = 5.969
  dimension "d301" = 5.969
  dimension "d302" = 5.969
  constraint coincident L12.end L13.start
  constraint perpendicular L13 L20
  constraint parallel L12 L21
  constraint parallel L12 L22
  constraint coincident L12 L23.end
  constraint parallel L12 L24
  constraint parallel L12 L25
  constraint parallel L12 L26
  constraint coincident L12 L27.end
  constraint parallel L12 L27
  constraint coincident L1.end L2.start
  constraint coincident L2 L28.end
  constraint coincident L2 L29.end
  constraint coincident L2 L30.end
  constraint coincident L2 L31.end
  constraint parallel L2 L32
  constraint coincident L2 L33.end
  constraint parallel L2 L34
  constraint parallel L2 L35
  constraint horizontal L36
  constraint vertical L37
  constraint horizontal L38
  constraint vertical L39
  constraint horizontal L40
  constraint vertical L41
  constraint horizontal L42
  constraint vertical L43
  constraint horizontal L44
  constraint vertical L45
  constraint horizontal L46
  constraint vertical L47
  constraint horizontal L48
  constraint vertical L49
  constraint horizontal L50
  constraint vertical L51
  constraint horizontal L52
  constraint vertical L53
  constraint horizontal L54
  constraint vertical L55
  constraint horizontal L56
  constraint vertical L57
  constraint horizontal L58
  constraint vertical L59
  constraint horizontal L60
  constraint vertical L61
  constraint horizontal L62
  constraint vertical L63
  constraint horizontal L64
  constraint vertical L65
  constraint horizontal L66
  constraint vertical L67
  constraint horizontal L68
  constraint vertical L69
  constraint horizontal L70
  constraint vertical L71
  constraint horizontal L72
  constraint vertical L73
  constraint horizontal L74
  constraint vertical L75
  constraint horizontal L76
  constraint vertical L77
  constraint horizontal L78
  constraint vertical L79
  constraint horizontal L80
  constraint vertical L81
  constraint horizontal L82
  constraint vertical L83
  constraint horizontal L84
  constraint vertical L85
  constraint horizontal L86
  constraint vertical L87
  constraint horizontal L88
  constraint vertical L89
  constraint horizontal L90
  constraint vertical L91
  constraint horizontal L92
  constraint vertical L93
  constraint horizontal L94
  constraint vertical L95
  constraint horizontal L96
  constraint vertical L97
  constraint horizontal L98
  constraint vertical L99
  measures "d256" distance of L12.end L20.end
  measures "d257" distance of L20.end L21.end
  measures "d258" distance of L21.end L22.end
  measures "d259" distance of L22.end L23.end
  measures "d260" distance of L23.end L24.end
  measures "d261" distance of L24.end L25.end
  measures "d262" distance of L25.end L26.end
  measures "d263" distance of L1.end L28.end
  measures "d264" distance of L28.end L29.end
  measures "d265" distance of L29.end L30.end
  measures "d266" distance of L30.end L31.end
  measures "d267" distance of L31.end L32.end
  measures "d268" distance of L32.end L33.end
  measures "d269" distance of L33.end L34.end
  measures "d270" distance of L34.end L35.end
  measures "d271" distance of L28.end L36.end
  measures "d272" distance of L28.end L38.end
  measures "d273" distance of L29.end L40.end
  measures "d274" distance of L29.end L42.end
  measures "d275" distance of L30.end L44.end
  measures "d276" distance of L30.end L46.end
  measures "d277" distance of L31.end L48.end
  measures "d278" distance of L31.end L50.end
  measures "d279" distance of L32.end L52.end
  measures "d280" distance of L32.end L54.end
  measures "d281" distance of L33.end L56.end
  measures "d282" distance of L33.end L58.end
  measures "d283" distance of L35.end L60.end
  measures "d284" distance of L35.end L62.end
  measures "d285" distance of L34.end L64.end
  measures "d286" distance of L34.end L66.end
  measures "d287" distance of L27.end L68.end
  measures "d288" distance of L27.end L70.end
  measures "d289" distance of L26.end L72.end
  measures "d290" distance of L26.end L74.end
  measures "d291" distance of L25.end L76.end
  measures "d292" distance of L25.end L78.end
  measures "d293" distance of L24.end L80.end
  measures "d294" distance of L24.end L82.end
  measures "d295" distance of L23.end L84.end
  measures "d296" distance of L23.end L86.end
  measures "d297" distance of L22.end L88.end
  measures "d298" distance of L22.end L90.end
  measures "d299" distance of L21.end L92.end
  measures "d300" distance of L21.end L94.end
  measures "d301" distance of L20.end L96.end
  measures "d302" distance of L20.end L98.end
extrude "Extrude12" cut sketch "Sketch30" against normal up to surface (5.969 mm away) contours L2 L36 L37 L38 L39 | L2 L40 L41 L42 L43 | L2 L44 L45 L46 L47 | L12 L96 L97 L98 L99 | L2 L48 L49 L50 L51 | L12 L92 L93 L94 L95 | L2 L52 L53 L54 L55 | L12 L88 L89 L90 L91 | L2 L56 L57 L58 L59 | L12 L84 L85 L86 L87 | L2 L64 L65 L66 L67 | L12 L80 L81 L82 L83 | L2 L60 L61 L62 L63 | L12 L76 L77 L78 L79 | L12 L72 L73 L74 L75 | L12 L68 L69 L70 L71 bodies 4 in component "Component''"
sketch "Sketch31" plane through (0, 5.969, 0) normal (0, 1, 0) x (-1, 0, 0)
  arc A0 (-495.3, 367.5922) -> (-596.1922, 266.7) centre (-482.6, 254) ccw
  line L0 (-596.1922, 266.7) -> (-602.5797, 266.7)
  arc A1 (-495.3, 373.9797) -> (-602.5797, 266.7) centre (-482.6, 254) ccw
  line L1 (-495.3, 373.9797) -> (-495.3, 367.5922)
  arc A2 (-469.9, 166.0118) -> (-394.6118, 241.3) centre (-482.6, 254) ccw
  line L2 (-394.6118, 241.3) -> (-388.2005, 241.3)
  arc A3 (-469.9, 159.6005) -> (-388.2005, 241.3) centre (-482.6, 254) ccw
  line L3 (-469.9, 159.6005) -> (-469.9, 166.0118)
  arc A4 (-420.383, 266.7) -> (-469.9, 316.217) centre (-482.6, 254) ccw
  line L4 (-469.9, 316.217) -> (-469.9, 322.6857)
  arc A5 (-413.9142, 266.7) -> (-469.9, 322.6857) centre (-482.6, 254) ccw
  line L5 (-413.9142, 266.7) -> (-420.383, 266.7)
  arc A6 (-469.9, 191.783) -> (-420.383, 241.3) centre (-482.6, 254) ccw
  line L6 (-420.383, 241.3) -> (-413.9142, 241.3)
  arc A7 (-469.9, 185.3142) -> (-413.9142, 241.3) centre (-482.6, 254) ccw
  line L7 (-469.9, 185.3142) -> (-469.9, 191.783)
  arc A8 (-394.6118, 266.7) -> (-469.9, 341.9882) centre (-482.6, 254) ccw
  line L8 (-469.9, 341.9882) -> (-469.9, 348.3995)
  arc A9 (-388.2005, 266.7) -> (-469.9, 348.3995) centre (-482.6, 254) ccw
  line L9 (-388.2005, 266.7) -> (-394.6118, 266.7)
  arc A10 (-469.9, 140.4077) -> (-369.0077, 241.3) centre (-482.6, 254) ccw
  line L10 (-369.0077, 241.3) -> (-362.6203, 241.3)
  arc A11 (-469.9, 134.0203) -> (-362.6203, 241.3) centre (-482.6, 254) ccw
  line L11 (-469.9, 134.0203) -> (-469.9, 140.4077)
  arc A12 (-369.0077, 266.7) -> (-469.9, 367.5922) centre (-482.6, 254) ccw
  line L12 (-469.9, 367.5922) -> (-469.9, 373.9797)
  arc A13 (-362.6203, 266.7) -> (-469.9, 373.9797) centre (-482.6, 254) ccw
  line L13 (-362.6203, 266.7) -> (-369.0077, 266.7)
  arc A14 (-570.5882, 241.3) -> (-495.3, 166.0118) centre (-482.6, 254) ccw
  line L14 (-495.3, 166.0118) -> (-495.3, 159.6005)
  arc A15 (-576.9995, 241.3) -> (-495.3, 159.6005) centre (-482.6, 254) ccw
  line L15 (-576.9995, 241.3) -> (-570.5882, 241.3)
  arc A16 (-495.3, 316.217) -> (-544.817, 266.7) centre (-482.6, 254) ccw
  line L16 (-544.817, 266.7) -> (-551.2857, 266.7)
  arc A17 (-495.3, 322.6857) -> (-551.2857, 266.7) centre (-482.6, 254) ccw
  line L17 (-495.3, 322.6857) -> (-495.3, 316.217)
  arc A18 (-544.817, 241.3) -> (-495.3, 191.783) centre (-482.6, 254) ccw
  line L18 (-495.3, 191.783) -> (-495.3, 185.3142)
  arc A19 (-551.2857, 241.3) -> (-495.3, 185.3142) centre (-482.6, 254) ccw
  line L19 (-551.2857, 241.3) -> (-544.817, 241.3)
  arc A20 (-495.3, 341.9882) -> (-570.5882, 266.7) centre (-482.6, 254) ccw
  line L20 (-570.5882, 266.7) -> (-576.9995, 266.7)
  arc A21 (-495.3, 348.3995) -> (-576.9995, 266.7) centre (-482.6, 254) ccw
  line L21 (-495.3, 348.3995) -> (-495.3, 341.9882)
  arc A22 (-596.1922, 241.3) -> (-495.3, 140.4077) centre (-482.6, 254) ccw
  line L22 (-495.3, 140.4077) -> (-495.3, 134.0203)
  arc A23 (-602.5797, 241.3) -> (-495.3, 134.0203) centre (-482.6, 254) ccw
  line L23 (-602.5797, 241.3) -> (-596.1922, 241.3)
  circle A24 centre (-482.6, 254) radius 152.4
  line L24 (-511.175, 251.0155) -> (-521.335, 251.0155)
  line L25 (-521.335, 251.0155) -> (-521.335, 256.9845)
  arc A25 (-485.5845, 282.575) -> (-521.335, 256.9845) centre (-493.2439, 255.508) ccw
  line L26 (-485.5845, 282.575) -> (-485.5845, 292.735)
  line L27 (-485.5845, 292.735) -> (-479.6155, 292.735)
  arc A26 (-454.025, 256.9845) -> (-479.6155, 292.735) centre (-481.092, 264.6439) ccw
  line L28 (-454.025, 256.9845) -> (-442.595, 256.9845)
  line L29 (-442.595, 256.9845) -> (-442.595, 251.0155)
  arc A27 (-479.6155, 225.425) -> (-442.595, 251.0155) centre (-472.206, 254.2792) ccw
  line L30 (-479.6155, 225.425) -> (-479.6155, 215.265)
  line L31 (-479.6155, 215.265) -> (-485.5845, 215.265)
  arc A28 (-511.175, 251.0155) -> (-485.5845, 215.265) centre (-484.108, 243.3561) ccw
sketch "Sketch32" plane through (0, 5.969, 0) normal (0, 1, 0) x (-1, 0, 0)
  circle A0 centre (0, 0) radius 152.4
  line L0 (2.9845, 88.9) -> (-2.9845, 88.9)
  line L1 (-2.9845, 88.9) -> (-2.9845, 114.3)
  line L2 (-2.9845, 114.3) -> (2.9845, 114.3)
  line L3 (2.9845, 114.3) -> (2.9845, 88.9)
  line L4 (-88.9, -2.9845) -> (-114.3, -2.9845)
  line L5 (-114.3, -2.9845) -> (-114.3, 2.9845)
  line L6 (-114.3, 2.9845) -> (-88.9, 2.9845)
  line L7 (-88.9, 2.9845) -> (-88.9, -2.9845)
  line L8 (2.9845, 2.9845) -> (38.1, 2.9845)
  line L9 (38.1, 2.9845) -> (38.1, -2.9845)
  line L10 (38.1, -2.9845) -> (2.9845, -2.9845)
  line L11 (2.9845, -2.9845) -> (2.9845, -38.1)
  line L12 (2.9845, -38.1) -> (-2.9845, -38.1)
  line L13 (-2.9845, -38.1) -> (-2.9845, -2.9845)
  line L14 (-2.9845, -2.9845) -> (-38.1, -2.9845)
  line L15 (-38.1, -2.9845) -> (-38.1, 2.9845)
  line L16 (-38.1, 2.9845) -> (-2.9845, 2.9845)
  line L17 (-2.9845, 2.9845) -> (-2.9845, 38.1)
  line L18 (-2.9845, 38.1) -> (2.9845, 38.1)
  line L19 (2.9845, 38.1) -> (2.9845, 2.9845)
  line L20 (114.3, -2.9845) -> (88.9, -2.9845)
  line L21 (88.9, -2.9845) -> (88.9, 2.9845)
  line L22 (88.9, 2.9845) -> (114.3, 2.9845)
  line L23 (114.3, 2.9845) -> (114.3, -2.9845)
  line L24 (2.9845, -114.3) -> (-2.9845, -114.3)
  line L25 (-2.9845, -114.3) -> (-2.9845, -88.9)
  line L26 (-2.9845, -88.9) -> (2.9845, -88.9)
  line L27 (2.9845, -88.9) -> (2.9845, -114.3)